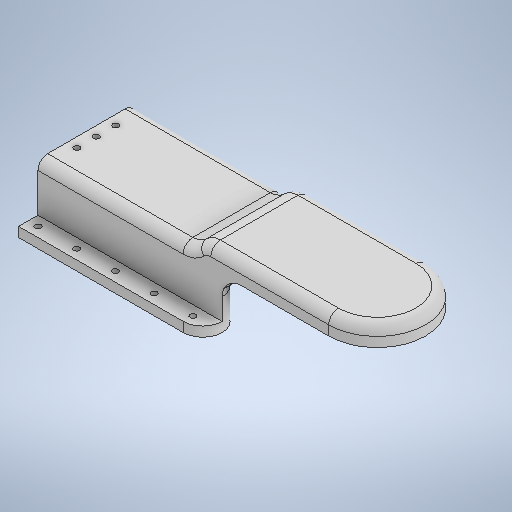
# Autodesk Inventor part: pulley_case_part_2_v2
Saved by Autodesk Inventor 2025 (Build 290162000, 162)
## iProperties
Created: 2025-02-05
Part Number: pulley_case_part_2_v2
Material: Generic
Document SubType Name: Modeling
Designer: danielrachi
Density: 1 g/cm^3
Appearance: Default
Author: danielrachi
Autodesk Inventor part; units mm, degrees
ref_plane "YZ Plane" through (0, 0, 0) normal (1, 0, 0) x (0, 1, 0)
ref_plane "XZ Plane" through (0, 0, 0) normal (0, 1, 0) x (-1, 0, 0)
ref_plane "XY Plane" through (0, 0, 0) normal (0, 0, 1) x (1, 0, 0)
sketch "Sketch1" plane through (0, 0, 0) normal (0, 0, 1) x (1, 0, 0)
  line L0 (-87.5, -18) -> (87.5, -18)
  line L1 (87.5, -18) -> (87.5, 18)
  line L2 (87.5, 18) -> (-87.5, 18)
  line L3 (-87.5, 18) -> (-87.5, -18)
  line L4 (-87.5, -18) -> (87.5, 18) construction
  line L5 (87.5, -18) -> (-87.5, 18) construction
  line L6 (-87.5, 18) -> (-7.5, 18)
  line L7 (-7.5, 18) -> (-7.5, 12)
  line L8 (-7.5, 12) -> (-87.5, 12)
  line L9 (-87.5, 12) -> (-87.5, 18)
  line L10 (87.5, -18) -> (7.5, -18)
  line L11 (7.5, -18) -> (7.5, 8)
  line L12 (7.5, 8) -> (87.5, 8)
  line L13 (87.5, 8) -> (87.5, -18)
  point P0 (0, 0)
  point P1 (-7.5, 18)
  point P2 (-87.5, 12)
  point P3 (7.5, -18)
  point P4 (72.5, 8)
  dimension "d2" = 80
  dimension "d4" = 80
  dimension "d5" = 26
  dimension "d62" = 15
  dimension "d63" = 160
  dimension "d68" = 10
  dimension "d69" = 30
  constraints: 28 end point, 6 parallel, 3 horizontal, 3 perpendicular, 2 midpoint, 1 point on line
  measures "d2" distance of L7.end L8.end
  measures "d4" distance of L11.end L12.end
  measures "d5" distance of L10.end L11.end
  measures "d62" distance of L12.end point (72.5, 8)
  measures "d63" distance from line of point (72.5, 8) L3
  measures "d68" distance between parallel lines of L2 L12
  measures "d69" distance between parallel lines of L0 L8
extrude "Extrusion1" add sketch "Sketch1" along normal blind 50 contours L3 L8 L7 L2 L1 L12 L11 L0
fillet "Fillet1" radius 10 3 edges at (-7.5, 18, 25) (-7.5, 12, 25) (7.5, 8, 25)
sketch "Sketch2" plane through (-87.5, -18, 0) normal (-1, 0, 0) x (0, 0, 1)
  line L0 (10, 0) -> (40, 0)
  line L1 (40, 0) -> (40, 20)
  line L2 (40, 20) -> (10, 20)
  line L3 (10, 20) -> (10, 0)
  line L4 (0, 30) -> (0, 0) projected
  line L5 (50, 30) -> (50, 0) projected
  line L6 (0, 0) -> (50, 0) projected
  line L7 (0, 30) -> (50, 30) projected
  point P0 (0, 18)
  dimension "d9" = 10
  dimension "d10" = 10
  dimension "d11" = 10
  constraints: 8 end point, 2 parallel, 1 collinear, 1 horizontal, 1 perpendicular
  measures "d9" distance between parallel lines of L3 L4
  measures "d10" distance between parallel lines of L5 L1
  measures "d11" distance between parallel lines of L2 L7
extrude "Extrusion2" cut sketch "Sketch2" against normal through all contours L3 L2 L1 L0
sketch "Sketch3" plane through (87.5, 8, 0) normal (0, -1, 0) x (1, 0, 0)
  circle A0 centre (-15, 25) radius 10.1
  line L0 (0, 0) -> (0, 50) projected
  circle A1 centre (-15, 25) radius 15
  point P0 (-87.5, 0)
  point P1 (0, 25)
  dimension "d14" = 20.2
  dimension "d15" = 30
  constraints: 2 centre point, 1 coincident, 1 horizontal alignment, 1 midpoint, 1 tangent
  measures "d14" diameter of A0
  measures "d15" diameter of A1
extrude "Extrusion3" cut sketch "Sketch3" against normal blind 6 contours A0
sketch "Sketch4" plane through (-87.5, -18, 0) normal (0, -1, 0) x (1, 0, 0)
  line L0 (0, 50) -> (95, 50) projected
  line L1 (0, 50) -> (95, 50)
  line L2 (95, 50) -> (95, 60)
  line L3 (95, 60) -> (0, 60)
  line L4 (0, 60) -> (0, 50)
  line L5 (95, 40) -> (95, 50) projected
  line L6 (0, 0) -> (0, 50) projected
  line L7 (0, 25) -> (90, 25)
  circle A0 centre (5, 55) radius 1.55
  circle A1 centre (25, 55) radius 1.55
  circle A2 centre (45, 55) radius 1.55
  circle A3 centre (65, 55) radius 1.55
  circle A4 centre (85, 55) radius 1.55
  line L8 (0, 0) -> (95, 0)
  line L9 (0, 0) -> (95, 0)
  line L10 (95, 0) -> (95, -10)
  line L11 (95, -10) -> (0, -10)
  line L12 (0, -10) -> (0, 0)
  circle A5 centre (5, -5) radius 1.55
  circle A6 centre (25, -5) radius 1.55
  circle A7 centre (45, -5) radius 1.55
  circle A8 centre (65, -5) radius 1.55
  circle A9 centre (85, -5) radius 1.55
  line L13 (0, 0) -> (95, 0)
  line L14 (0, 0) -> (95, 0)
  line L15 (95, 0) -> (95, -10)
  line L16 (95, -10) -> (0, -10)
  line L17 (0, -10) -> (0, 0)
  circle A10 centre (5, -5) radius 1.55
  circle A11 centre (25, -5) radius 1.55
  circle A12 centre (45, -5) radius 1.55
  circle A13 centre (65, -5) radius 1.55
  circle A14 centre (85, -5) radius 1.55
  point P0 (87.5, 0)
  point P1 (0, 55)
  point P2 (0, -5)
  dimension "d18" = 10
  dimension "d19" = 3.1
  dimension "d20" = 5
  dimension "d23" = 20
  constraints: 30 end point, 17 symmetric about line, 15 centre point, 3 horizontal, 2 midpoint, 2 parallel, 1 collinear, 1 horizontal alignment, 1 perpendicular, 18 other
  measures "d18" distance of L2.end L1.end
  measures "d19" diameter of A0
  measures "d20" distance from line of L4 A0.centre
  measures "d23" distance of A0.centre A1.centre
extrude "Extrusion4" add sketch "Sketch4" against normal blind 5
sketch "Sketch9" plane through (-87.5, 12, 0) normal (-1, 0, 0) x (0, 0, 1)
  line L0 (4.9, -30) -> (45.1, -30)
  line L1 (45.1, -30) -> (45.1, -4.9)
  line L2 (45.1, -4.9) -> (4.9, -4.9)
  line L3 (4.9, -4.9) -> (4.9, -30)
  line L4 (40, -30) -> (60, -30) projected
  line L5 (10, -30) -> (10, -10) projected
  line L6 (40, -10) -> (40, -30) projected
  line L7 (10, -10) -> (40, -10) projected
  point P0 (0, -12)
  point P1 (40, -30)
  dimension "d44" = 5.1
  dimension "d45" = 5.1
  dimension "d46" = 5.1
  constraints: 8 end point, 2 parallel, 1 collinear, 1 horizontal, 1 perpendicular
  measures "d44" distance between parallel lines of L3 L5
  measures "d45" distance between parallel lines of L1 L6
  measures "d46" distance between parallel lines of L2 L7
extrude "Extrusion7" cut sketch "Sketch9" against normal blind 10 contours L3 L2 L1 L0 L6 L7 L5
sketch "Sketch11" plane through (-87.5, 7.1, 4.9) normal (0, -1, 0) x (1, 0, 0)
  circle A0 centre (5, 10) radius 1.55
  line L0 (10, 0) -> (0, 0) projected
  line L1 (0, 40.2) -> (10, 40.2) projected
  line L2 (10, 0) -> (10, 40.2)
  circle A1 centre (5, 20) radius 1.55
  circle A2 centre (5, 30) radius 1.55
  point P0 (87.5, -4.9)
  point P1 (5, 0)
  dimension "d50" = 3.1
  dimension "d51" = 10
  dimension "d54" = 10
  constraints: 3 centre point, 2 end point, 2 vertical, 1 midpoint, 1 vertical alignment, 4 other
  measures "d50" diameter of A0
  measures "d51" distance from line of L0 A0.centre
  measures "d54" distance of A0.centre A1.centre
fillet "Fillet2" radius 25 2 edges at (87.5, 13, 50) (87.5, 13, 0)
extrude "Extrusion8" cut sketch "Sketch11" against normal blind 10
fillet "Fillet3" radius 10 2 edges at (7.5, -15.5, 60) (7.5, -15.5, -10)
fillet "Fillet4" radius 5 7 edges at (-2.2078, 17.2195, 50) (-50.0589, 12, 50) (80.1777, 18, 42.6777) (32.0826, 18, 0) (-2.2078, 17.2195, 0) (-50.0589, 12, 0) (32.0826, 18, 50)
fillet "Fillet6" radius 10 2 edges at (7.5, -10, 10) (7.5, -10, 40)
equation "\"screw_out_width\" = 7.5"
body "Solid1"
